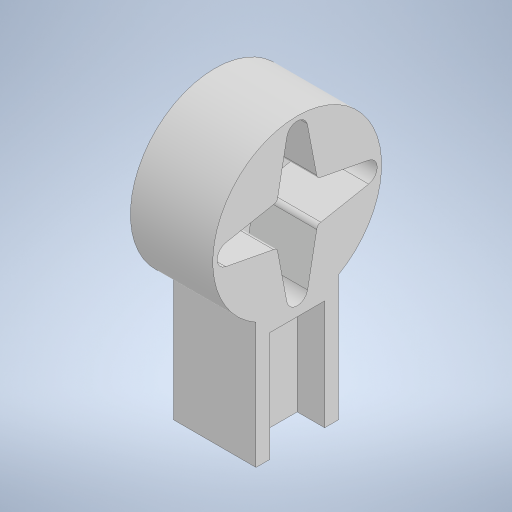
# Autodesk Inventor part: Part_3_hand
Saved by Autodesk Inventor 2023 (Build 270158000, 158)
## iProperties
Created: 2023-09-29
Part Number: Part_3_hand
Material: Generic
Document SubType Name: Modeling
Designer: zskus
Density: 1 g/cm^3
Appearance: Default
Author: zskus
Autodesk Inventor part; units mm, degrees
ref_plane "YZ Plane" through (0, 0, 0) normal (1, 0, 0) x (0, 1, 0)
ref_plane "XZ Plane" through (0, 0, 0) normal (0, 1, 0) x (-1, 0, 0)
ref_plane "XY Plane" through (0, 0, 0) normal (0, 0, 1) x (1, 0, 0)
sketch "Sketch1" plane through (0, 0, 0) normal (1, 0, 0) x (0, 1, 0)
  line L0 (0, 9.525) -> (-50.8, 9.525)
  line L1 (-50.8, 9.525) -> (-50.8, -9.525)
  line L2 (-50.8, -9.525) -> (0, -9.525)
  line L3 (0, -9.525) -> (0, 9.525)
  arc A0 (0, -9.525) -> (0, 9.525) centre (0, 0) ccw
  dimension "d0" = 19.05
  dimension "d1" = 50.8
  constraints: 8 end point, 2 parallel, 2 point on circle, 2 tangent, 1 centre point, 1 coincident, 1 horizontal, 1 perpendicular
  measures "d0" distance between parallel lines of L2 L0
  measures "d1" distance of L1.end L2.end
extrude "Extrusion1" add sketch "Sketch1" along normal blind 19.05
sketch "Sketch3" plane through (19.05, 0, 0) normal (1, 0, 0) x (0, 0, -1)
  line L0 (-9.525, 0) -> (-9.525, -50.8) projected
  line L1 (-9.525, -50.8) -> (9.525, -50.8) projected
  line L2 (9.525, -50.8) -> (9.525, 0) projected
  arc A0 (9.525, 0) -> (-9.525, 0) centre (0, 0) ccw projected
  line L3 (-6.35, -50.8) -> (6.35, -50.8)
  line L4 (6.35, -50.8) -> (6.35, -25.4)
  line L5 (6.35, -25.4) -> (-6.35, -25.4)
  line L6 (-6.35, -25.4) -> (-6.35, -50.8)
  point P0 (0, -50.8)
  dimension "d18" = 12.7
  dimension "d19" = 6.35
  dimension "d20" = 25.4
  constraints: 8 end point, 2 parallel, 1 horizontal, 1 midpoint, 1 perpendicular, 1 point on line
  measures "d18" distance of L4.end L5.end
  measures "d19" distance from line of point (0, -50.8) L6
  measures "d20" distance between parallel lines of L1 L5
extrude "Extrusion3" cut sketch "Sketch3" against normal blind 6.35 contours L6 L5 L4 L1
sketch "Sketch4" plane through (19.05, 0, 0) normal (1, 0, 0) x (0, 0, -1)
  line L0 (-6.35, -50.8) -> (-6.35, -25.4) projected
  line L1 (-6.35, -25.4) -> (6.35, -25.4) projected
  line L2 (6.35, -25.4) -> (6.35, -50.8) projected
  line L3 (6.35, -50.8) -> (9.525, -50.8) projected
  line L4 (9.525, -50.8) -> (9.525, 0) projected
  arc A0 (9.525, 0) -> (-9.525, 0) centre (0, 0) ccw projected
  line L5 (-9.525, 0) -> (-9.525, -50.8) projected
  line L6 (-9.525, -50.8) -> (-6.35, -50.8) projected
  circle A1 centre (0, 0) radius 9.525
  line L7 (-14.2875, 12.7) -> (12.7, 12.7)
  line L8 (12.7, 12.7) -> (12.7, -4.7625)
  line L9 (12.7, -4.7625) -> (-14.2875, -4.7625)
  line L10 (-14.2875, -4.7625) -> (-14.2875, 12.7)
  point P0 (-8.2489, -4.7625)
  point P1 (-9.525, 0)
  point P2 (9.525, 0)
  point P3 (8.2489, -4.7625)
  dimension "d28" = 19.05
  constraints: 8 end point, 2 parallel, 1 centre point, 1 horizontal, 1 perpendicular
  measures "d28" diameter of A1
extrude "Extrusion4" [suppressed]
sketch "Sketch5" plane through (19.05, 0, 0) normal (1, 0, 0) x (0, 0, -1)
  arc A0 (1.8331, 11.9745) -> (-1.9, 11.7198) centre (0, 11.3568) ccw
  line L0 (-1.9, 11.7198) -> (-4, 0.7283)
  arc A1 (-5.4371, -0.709) -> (-4, 0.7283) centre (-5.4371, 0.7281) ccw
  line L1 (-5.4371, -0.709) -> (-16.4286, -2.8088)
  arc A2 (-16.4286, -2.8088) -> (-16.4286, -6.6088) centre (-16.0656, -4.7088) ccw
  line L2 (-16.4286, -6.6088) -> (-5.4371, -8.7087)
  arc A3 (-4, -10.146) -> (-5.4371, -8.7087) centre (-5.4371, -10.1458) ccw
  line L3 (-4, -10.146) -> (-1.9, -21.1375)
  arc A4 (-1.9, -21.1375) -> (1.9, -21.1375) centre (0, -20.7745) ccw
  line L4 (1.9, -21.1375) -> (4, -10.146)
  arc A5 (5.4371, -8.7088) -> (4, -10.146) centre (5.4371, -10.146) ccw
  line L5 (5.4371, -8.7088) -> (16.4286, -6.6088)
  arc A6 (16.4286, -6.6088) -> (16.4286, -2.8088) centre (16.0656, -4.7088) ccw
  line L6 (16.4286, -2.8088) -> (5.4367, -0.7088)
  arc A7 (4.0053, 0.6052) -> (5.4367, -0.7088) centre (5.4371, 0.7283) ccw
  line L7 (4.0053, 0.6052) -> (1.8331, 11.9745)
  line L8 (-6.35, -50.8) -> (-6.35, -25.4) projected
  line L9 (-6.35, -25.4) -> (6.35, -25.4) projected
  line L10 (6.35, -25.4) -> (6.35, -50.8) projected
  line L11 (6.35, -50.8) -> (9.525, -50.8) projected
  line L12 (9.525, -50.8) -> (9.525, 0) projected
  arc A8 (9.525, 0) -> (-9.525, 0) centre (0, 0) ccw projected
  line L13 (-9.525, 0) -> (-9.525, -50.8) projected
  line L14 (-9.525, -50.8) -> (-6.35, -50.8) projected
  line L15 (-4.509, 0.7712) -> (-2.399, 11.8152)
  arc A9 (2.3259, 12.1019) -> (-2.399, 11.8152) centre (0, 11.3568) ccw
  line L16 (2.3259, 12.1019) -> (4.5097, 0.672)
  arc A10 (4.5097, 0.672) -> (5.4797, -0.1998) centre (5.4371, 0.7283) ccw
  line L17 (5.4797, -0.1998) -> (16.524, -2.3098)
  arc A11 (16.524, -7.1078) -> (16.524, -2.3098) centre (16.0656, -4.7088) ccw
  line L18 (16.524, -7.1078) -> (5.48, -9.2178)
  arc A12 (5.48, -9.2178) -> (4.509, -10.1889) centre (5.4371, -10.146) ccw
  line L19 (4.509, -10.1889) -> (2.399, -21.2328)
  arc A13 (-2.399, -21.2328) -> (2.399, -21.2328) centre (0, -20.7745) ccw
  line L20 (-2.399, -21.2328) -> (-4.509, -10.1888)
  arc A14 (-4.509, -10.1888) -> (-5.48, -9.2177) centre (-5.4371, -10.1458) ccw
  line L21 (-5.48, -9.2177) -> (-16.524, -7.1078)
  arc A15 (-16.524, -2.3098) -> (-16.524, -7.1078) centre (-16.0656, -4.7088) ccw
  line L22 (-16.524, -2.3098) -> (-5.48, -0.2)
  arc A16 (-5.48, -0.2) -> (-4.509, 0.7712) centre (-5.4371, 0.7281) ccw
  circle A17 centre (0, -4.7088) radius 19.5082
  point P0 (2.905, 9.0712)
  point P1 (9.525, -0.9727)
  point P2 (9.525, -8.445)
  point P3 (9.525, -21.7336)
  point P4 (-9.525, -21.7336)
  point P5 (-9.525, -8.4449)
  point P6 (-9.525, -0.9728)
  point P7 (-2.9244, 9.065)
  dimension "d29" = 0
  dimension "d30" = 0.508
  constraints: 32 end point, 32 point on circle, 17 centre point, 1 coincident, 15 other
  measures "d29" horizontal distance of A8.centre A0.centre
  measures "d30" distance between parallel lines of L0 L15
extrude "Extrusion5" add sketch "Sketch5" against normal up to surface (19.05 mm away) contours L7 A8 L0 A0 | A0 L0 A8 L15 A9 L16 L7 | A8 L16 A10 L17 L12 L6 A7 L7 | L7 A7 L6 L12 L5 A5 L4 A4 L3 A3 L2 L13 L1 A1 L0 A8 | L0 A1 L1 L13 L22 A16 L15 A8 | L16 A9 L15 A8 L13 L22 A15 L21 A17 L12 L18 A11 L17 | L12 L17 A11 L18 L5 A6 L6 | L6 A6 L5 L12 | L13 L2 A2 L1 | L1 A2 L2 L13 L21 A15 L22 | L12 L18 A12 L19 A13 L20 A14 L21 L13 L2 A3 L3 A4 L4 A5 L5
extrude "Extrusion6" cut sketch "Sketch5" against normal blind 14.2875 contours L7 A8 L0 A0 | A0 L0 A8 L15 A9 L16 L7 | A8 L16 A10 L17 L12 L6 A7 L7 | L7 A7 L6 L12 L5 A5 L4 A4 L3 A3 L2 L13 L1 A1 L0 A8 | L0 A1 L1 L13 L22 A16 L15 A8 | L12 L17 A11 L18 L5 A6 L6 | L6 A6 L5 L12 | L13 L2 A2 L1 | L1 A2 L2 L13 L21 A15 L22 | L12 L18 A12 L19 A13 L20 A14 L21 L13 L2 A3 L3 A4 L4 A5 L5
equation "\"d19\" = 0.5 * d18"
body "Solid1"
